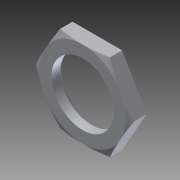
# Autodesk Inventor part: AT503M
Saved by Autodesk Inventor 2011 SP1 (Build 150282100, 282)
## iProperties
Created: 2013-12-24
Part Number: AT503M
Catalog Web Link: www.cadenas.de
Description: Hex Face Nut - Bushing Mount Miniature Toggles-Series M - Standard Hardwarw for Small & Large Bushings
Vendor: NKKSWITCHES
Document SubType Name: Modeling
Designer: PARTuser1
Manufacturer: NKKSWITCHES
Density: 1 g/cm^3
Category: PARTsolutions
Company: NKKSWITCHES
Title: AT503M
Author: Cadenas PARTsolutions
Comments: Series M - Standard Hardwarw for Small & Large Bushings
PSOL_IDENT_0: {$CADENAS_DATA\23d-libs\nkkswitches\toggle\m\hardware\hex_face_nut.prj},194 {VTYP=3D},{NB=AT503M},{L
PSOL_IDENT_1: INA=AT503M},{NN=Hex Face Nut - Bushing Mount Miniature Toggles},{DATE=07.12.2009 12:30:45},{GEOMDATE
PSOL_IDENT_2: =07.12.2009 11:50:00},{VERSION=},{LINEID=10},{LINESUBID=-1},{WBVAR=}  {NB=AT503M},{LINA=AT503M},{KT=
PSOL_IDENT_3: DUMMY},{PN=AT503M},{S=0.551},{D=M12},{DMAX=0.472},{DMIN=0.430},{T=0.094},{W=0.630}
CNS_NN: Hex Face Nut - Bushing Mount Miniature Toggles
CNS_NT: Series M - Standard Hardwarw for Small & Large Bushings
CNS_NB: AT503M
CNS_NBSYN: $PN.
CNS_LINA: AT503M
CNS_PN: AT503M
CNS_S: 0.551
CNS_D: M12
CNS_DMAX: 0.472
CNS_DMIN: 0.430
CNS_T: 0.094
CNS_W: 0.630
SUPPLIER: NKKSWITCHES
ARTICLENO: AT503M
BOMINFO: AT503M
CREATOR: CADENAS GmbH
Autodesk Inventor part; units mm, degrees
sketch "Sketch_1" plane through (0, 0, 0) normal (1, 0, 0) x (0, 1, 0)
  line L0 (0, -1.1938) -> (0, 1.1938)
  line L1 (0, 1.1938) -> (6.9977, 1.1938)
  line L2 (6.9977, 1.1938) -> (8.3972, 0.6844)
  line L3 (8.3972, 0.6844) -> (8.3972, -1.1938)
  line L4 (8.3972, -1.1938) -> (0, -1.1938)
  line L5 (0, -1.1938) -> (0, 1.1938)
  constraints: 12 end point
revolve "Revolution1" add sketch "Sketch_1" angle 360 about axis through (0, 0, -1.1938) along (0, 0, -1)
sketch "Sketch_2" plane through (0, 0, 0) normal (0, 0, 1) x (1, 0, 0)
  line L0 (-13.9954, 13.9954) -> (-13.9954, -13.9954)
  line L1 (-13.9954, -13.9954) -> (13.9954, -13.9954)
  line L2 (13.9954, -13.9954) -> (13.9954, 13.9954)
  line L3 (13.9954, 13.9954) -> (-13.9954, 13.9954)
  line L4 (-8.001, 0) -> (-4.0401, -6.9977)
  line L5 (-4.0401, -6.9977) -> (4.0401, -6.9977)
  line L6 (4.0401, -6.9977) -> (8.001, 0)
  line L7 (8.001, 0) -> (4.0401, 6.9977)
  line L8 (4.0401, 6.9977) -> (-4.0401, 6.9977)
  line L9 (-4.0401, 6.9977) -> (-8.001, 0)
  constraints: 20 end point
extrude "Extrusion1" cut sketch "Sketch_2" along normal mid plane 4.7752
sketch "Sketch3" plane through (4.0401, 6.9977, -1.1938) normal (0, 0, -1) x (-1, 0, 0)
  point P0 (4.0401, -6.9977)
hole "Drilling 1" at (0, 0, -1.1938) direction (0, 0, 1) diameter 10.106 depth 2.3876 countersink diameter 11.9888 countersink angle 90
ref_plane "nut_XY" through (0, 0, -1.1938) normal (0, 0, 1) x (1, 0, 0)
ref_plane "nut_YZ" through (0, 0, -1.1938) normal (1, 0, 0) x (0, 1, 0)
ref_plane "nut_ZX" through (0, 0, -1.1938) normal (0, 1, 0) x (0, 0, 1)
body "Solid1"
